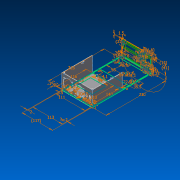
# Autodesk Inventor part: case
Saved by Autodesk Inventor 2015 (Build 190159000, 159)
## iProperties
Created: 2017-03-22
Part Number: case
Material: Generic
Document SubType Name: Modeling
Designer: ZigZagJoe
Density: 1 g/cm^3
Appearance: Default
Author: ZigZagJoe
Autodesk Inventor part; units mm, degrees
ref_plane "YZ Plane" through (0, 0, 0) normal (1, 0, 0) x (0, 1, 0)
ref_plane "XZ Plane" through (0, 0, 0) normal (0, 1, 0) x (-1, 0, 0)
ref_plane "XY Plane" through (0, 0, 0) normal (0, 0, 1) x (1, 0, 0)
sketch "Case Bottom" plane through (0, 0, 0) normal (0, 1, 0) x (-1, 0, 0)
  line L0 (18.5751, 111.0627) -> (-98.4249, 111.0627)
  line L1 (-98.4249, 111.0627) -> (-98.4249, -118.9373)
  line L2 (-98.4249, -118.9373) -> (18.5751, -118.9373)
  line L3 (18.5751, -118.9373) -> (18.5751, 111.0627)
  line L4 (16.5751, 109.0627) -> (-96.4249, 109.0627)
  line L5 (-96.4249, 109.0627) -> (-96.4249, -116.9373)
  line L6 (-96.4249, -116.9373) -> (16.5751, -116.9373)
  line L7 (16.5751, -116.9373) -> (16.5751, 109.0627)
  line L8 (-95.9249, 108.0627) -> (15.0751, 108.0627)
  line L9 (15.0751, 108.0627) -> (15.0751, -106.9373)
  line L10 (15.0751, -106.9373) -> (-95.9249, -106.9373)
  line L11 (-95.9249, -106.9373) -> (-95.9249, 108.0627)
  line L12 (-25.9249, 68.0627) -> (-84.9249, 68.0627)
  line L13 (-84.9249, 68.0627) -> (-84.9249, 15.0627)
  line L14 (-84.9249, 15.0627) -> (-25.9249, 15.0627)
  line L15 (-25.9249, 15.0627) -> (-25.9249, 68.0627)
  line L16 (18.5751, -4.9373) -> (-98.4249, -4.9373)
  line L17 (15.0751, -31.9373) -> (-95.9249, -31.9373)
  circle A0 centre (8.0751, -54.4373) radius 3
  circle A1 centre (8.0751, -54.4373) radius 2.05
  circle A2 centre (-31.4249, -67.4373) radius 3
  circle A3 centre (-31.4249, -67.4373) radius 2.05
  circle A4 centre (-78.3249, -89.9373) radius 3
  circle A5 centre (-78.3249, -89.9373) radius 2.05
  circle A6 centre (-77.9249, -1.9373) radius 3
  circle A7 centre (-77.9249, -1.9373) radius 2.05
  circle A8 centre (8.0751, -4.9373) radius 3
  circle A9 centre (8.5751, 99.0627) radius 3
  circle A10 centre (8.5751, 99.0627) radius 2.05
  circle A11 centre (-33.4249, 100.0627) radius 3
  circle A12 centre (-33.4249, 100.0627) radius 2.05
  circle A13 centre (-88.9249, 82.0627) radius 3
  point P0 (0, 0)
  dimension "d1" = 230
  dimension "d2" = 113
  dimension "d3" = 2
  dimension "d4" = 2
  dimension "d5" = 2
  dimension "d6" = 2
  dimension "d77" = 0.5
  dimension "d78" = 111
  dimension "d79" = 1
  dimension "d129" = 59
  dimension "d130" = 53
  dimension "d131" = 11
  dimension "d132" = 40
  dimension "d181" = 116
  dimension "d200" = 215
  dimension "d201" = 140
  dimension "d202" = 6
  dimension "d203" = 4.1
  dimension "d204" = 22.5
  dimension "d205" = 7
  dimension "d206" = 6
  dimension "d207" = 4.1
  dimension "d208" = 64.5
  dimension "d210" = 35.5
  dimension "d211" = 6
  dimension "d212" = 4.1
  dimension "d213" = 17.6
  dimension "d214" = 58
  dimension "d215" = 6
  dimension "d216" = 4.1
  dimension "d218" = 18
  dimension "d219" = 110
  dimension "d220" = 6
  dimension "d272" = 117
  dimension "d317" = 6
  dimension "d318" = 4.1
  dimension "d319" = 6
  dimension "d320" = 4.1
  dimension "d321" = 6
  dimension "d322" = 26
  dimension "d323" = 7
  dimension "d324" = 62.5
  dimension "d325" = 8
  dimension "d326" = 104.5
  dimension "d327" = 9
  constraints: 36 end point, 14 centre point, 8 parallel, 6 coincident, 6 perpendicular, 5 point on line, 4 horizontal
  measures "d1" distance of L2.end L0.start
  measures "d2" distance of L4.start L4.end
  measures "d3" distance between parallel lines of L3 L7
  measures "d4" distance between parallel lines of L5 L1
  measures "d5" distance between parallel lines of L4 L0
  measures "d6" distance between parallel lines of L2 L6
  measures "d77" distance between parallel lines of L5 L11
  measures "d78" distance of L8.start L8.end
  measures "d79" distance between parallel lines of L8 L4
  measures "d129" distance of L14.end L13.end
  measures "d130" distance of L13.end L12.end
  measures "d131" distance between parallel lines of L11 L13
  measures "d132" distance between parallel lines of L8 L12
  measures "d181" distance between parallel lines of L0 L16
  measures "d200" distance between parallel lines of L10 L8
  measures "d201" distance between parallel lines of L17 L8
  measures "d202" diameter of A0
  measures "d203" diameter of A1
  measures "d204" distance from line of A0.centre L17
  measures "d205" distance from line of L9 A0.centre
  measures "d206" diameter of A2
  measures "d207" diameter of A3
  measures "d208" distance from line of A2.centre L11
  measures "d210" distance from line of A2.centre L17
  measures "d211" diameter of A4
  measures "d212" diameter of A5
  measures "d213" distance from line of L11 A4.centre
  measures "d214" distance from line of L17 A4.centre
  measures "d215" diameter of A6
  measures "d216" diameter of A7
  measures "d218" distance from line of L11 A6.centre
  measures "d219" distance from line of L8 A6.centre
  measures "d220" diameter of A8
  measures "d272" distance between parallel lines of L1 L3
  measures "d317" diameter of A9
  measures "d318" diameter of A10
  measures "d319" diameter of A11
  measures "d320" diameter of A12
  measures "d321" diameter of A13
  measures "d322" distance from line of L8 A13.centre
  measures "d323" distance from line of L11 A13.centre
  measures "d324" distance from line of L11 A11.centre
  measures "d325" distance from line of L8 A11.centre
  measures "d326" distance from line of L11 A9.centre
  measures "d327" distance from line of L8 A9.centre
extrude "Base" add sketch "Case Bottom" along normal blind 3 contours L3 L16 L7 L4 L5 L1 L0 | L3 L2 L1 L16 L5 L6 L7 | L16 L9 L8 L11 L5 L4 L7 | L7 L6 L5 L16 L11 L10 L9 | A6 | L16 A8 L11 L8 L9 | L9 L17 L11 L16 A8 | L9 L10 L11 L17 | A8 L16 | L16 A8 | L15 L14 L13 L12 | A0 | A1 | A2 | A3 | A4 | A5 | A7 | A9 | A10 | A11 | A12 | A13
extrude "Walls" add sketch "Case Bottom" against normal blind 58 contours L3 L16 L7 L4 L5 L1 L0 | L3 L2 L1 L16 L5 L6 L7
sketch "Front Panel" plane through (-18.5751, 3, 111.0627) normal (0, 0, 1) x (1, 0, 0)
  line L0 (113, -51.5) -> (73, -51.5)
  line L1 (73, -51.5) -> (73, -11.5)
  line L2 (73, -11.5) -> (113, -11.5)
  line L3 (113, -11.5) -> (113, -51.5)
  circle A0 centre (109, -47.5) radius 2
  circle A1 centre (77, -47.5) radius 2
  circle A2 centre (77, -15.5) radius 2
  circle A3 centre (109, -15.5) radius 2
  circle A4 centre (93, -31.5) radius 20
  circle A5 centre (109, -47.5) radius 4
  circle A6 centre (109, -15.5) radius 4
  circle A7 centre (77, -15.5) radius 4
  circle A8 centre (77, -47.5) radius 4
  line L4 (115, -3) -> (2, -3) projected
  line L5 (28, -46.875) -> (16, -46.875)
  line L6 (16, -46.875) -> (16, -15.875)
  line L7 (16, -15.875) -> (28, -15.875)
  line L8 (28, -15.875) -> (28, -46.875)
  line L9 (69, -51.5) -> (29, -51.5)
  line L10 (29, -51.5) -> (29, -11.5)
  line L11 (29, -11.5) -> (69, -11.5)
  line L12 (69, -11.5) -> (69, -51.5)
  circle A9 centre (22, -30.5) radius 3.625
  circle A10 centre (22, -39.125) radius 1.5
  circle A11 centre (22, -21.875) radius 1.5
  circle A12 centre (22, -45.375) radius 1.5
  line L13 (2.5, -6.5) -> (114.5, -6.5)
  line L14 (114.5, -6.5) -> (114.5, -7.5)
  line L15 (114.5, -7.5) -> (2.5, -7.5)
  line L16 (2.5, -7.5) -> (2.5, -6.5)
  line L17 (91.5, -9.3) -> (78.5, -9.3)
  line L18 (78.5, -9.3) -> (78.5, -3.3)
  line L19 (78.5, -3.3) -> (91.5, -3.3)
  line L20 (91.5, -3.3) -> (91.5, -9.3)
  line L21 (68.5, -8.7) -> (63.5, -8.7)
  line L22 (62.5, -7.7) -> (62.5, -4.7)
  line L23 (62.5, -4.7) -> (69.5, -4.7)
  line L24 (69.5, -4.7) -> (69.5, -7.7)
  arc A13 (68.5, -8.7) -> (69.5, -7.7) centre (68.5, -7.7) ccw
  arc A14 (62.5, -7.7) -> (63.5, -8.7) centre (63.5, -7.7) ccw
  circle A15 centre (12, -6.75) radius 0.6
  line L25 (115, -3) -> (115, -61) projected
  line L26 (2, -3) -> (2, -61) projected
  line L27 (15, -11.5) -> (2.5, -11.5)
  line L28 (2.5, -11.5) -> (2.5, -49.5)
  line L29 (2.5, -49.5) -> (15, -49.5)
  line L30 (15, -49.5) -> (15, -11.5)
  line L31 (117, -61) -> (0, -61) projected
  line L32 (0, 0) -> (117, 0) projected
  line L33 (12.25, -37.5) -> (5.25, -37.5)
  line L34 (5.25, -37.5) -> (5.25, -23.5)
  line L35 (5.25, -23.5) -> (12.25, -23.5)
  line L36 (12.25, -23.5) -> (12.25, -37.5)
  circle A16 centre (8.75, -45) radius 1.6
  circle A17 centre (8.75, -16) radius 1.6
  point P0 (18.5751, -3)
  point P1 (62.5, -8.7)
  dimension "d11" = 40
  dimension "d12" = 40
  dimension "d13" = 4
  dimension "d14" = 4
  dimension "d15" = 4
  dimension "d16" = 4
  dimension "d17" = 32
  dimension "d18" = 32
  dimension "d19" = 32
  dimension "d20" = 32
  dimension "d21" = 4
  dimension "d22" = 4
  dimension "d23" = 40
  dimension "d31" = 2
  dimension "d32" = 8.5
  dimension "d33" = 4
  dimension "d34" = 8
  dimension "d35" = 20
  dimension "d36" = 20
  dimension "d37" = 12
  dimension "d38" = 31
  dimension "d39" = 40
  dimension "d40" = 4
  dimension "d41" = 7.25
  dimension "d42" = 3
  dimension "d43" = 3
  dimension "d44" = 8.625
  dimension "d45" = 8.625
  dimension "d46" = 6
  dimension "d47" = 6
  dimension "d48" = 0
  dimension "d49" = 0
  dimension "d50" = 6
  dimension "d51" = 3
  dimension "d52" = 6.25
  dimension "d53" = 0
  dimension "d59" = 112
  dimension "d60" = 1
  dimension "d61" = 3.5
  dimension "d62" = 13
  dimension "d63" = 6
  dimension "d64" = 7
  dimension "d65" = 4
  dimension "d66" = 1.8
  dimension "d67" = 3.2
  dimension "d68" = 23
  dimension "d69" = 45
  dimension "d70" = 1
  dimension "d71" = 1.2
  dimension "d72" = 102.5
  dimension "d73" = 0.75
  dimension "d74" = 0.5
  dimension "d275" = 12.5
  dimension "d276" = 38
  dimension "d277" = 30.5
  dimension "d278" = 61
  dimension "d279" = 3.2
  dimension "d280" = 3.2
  dimension "d281" = 3.5
  dimension "d282" = 7
  dimension "d283" = 14
  dimension "d285" = 7.5
  dimension "d286" = 3.5
  dimension "d287" = 29
  constraints: 64 end point, 18 centre point, 16 parallel, 8 horizontal, 8 perpendicular, 8 tangent, 4 coincident, 4 point on circle, 2 point on line, 1 equal radius
  measures "d11" distance of L1.end L2.end
  measures "d12" distance of L0.end L1.end
  measures "d13" diameter of A0
  measures "d14" diameter of A1
  measures "d15" diameter of A2
  measures "d16" diameter of A3
  measures "d17" distance of A0.centre A3.centre
  measures "d18" distance of A1.centre A0.centre
  measures "d19" distance of A1.centre A2.centre
  measures "d20" distance of A3.centre A2.centre
  measures "d21" distance from line of L0 A0.centre
  measures "d22" distance from line of L3 A0.centre
  measures "d23" diameter of A4
  measures "d31" horizontal distance of L0.start L4.start
  measures "d32" distance between parallel lines of L4 L2
  measures "d33" distance from line of L1 A2.centre
  measures "d34" diameter of A7
  measures "d35" distance from line of L3 A4.centre
  measures "d36" distance from line of A4.centre L2
  measures "d37" distance of L6.end L7.end
  measures "d38" distance of L5.end L6.end
  measures "d39" distance of L10.end L11.end
  measures "d40" distance between parallel lines of L12 L1
  measures "d41" diameter of A9
  measures "d42" diameter of A10
  measures "d43" diameter of A11
  measures "d44" distance of A9.centre A11.centre
  measures "d45" distance of A9.centre A10.centre
  measures "d46" distance from line of L8 A9.centre
  measures "d47" distance from line of L6 A9.centre
  measures "d48" horizontal distance of A9.centre A10.centre
  measures "d49" horizontal distance of A9.centre A11.centre
  measures "d50" distance from line of L7 A11.centre
  measures "d51" diameter of A12
  measures "d52" distance of A12.centre A10.centre
  measures "d53" horizontal distance of A12.centre A10.centre
  measures "d59" distance of L14.end L15.end
  measures "d60" distance of L13.end L14.end
  measures "d61" distance between parallel lines of L4 L13
  measures "d62" distance of L18.end L19.end
  measures "d63" distance of L17.end L18.end
  measures "d64" distance of L22.end L23.end
  measures "d65" distance of point (62.5, -8.7) L22.end
  measures "d66" distance between parallel lines of L13 L23
  measures "d67" distance between parallel lines of L13 L19
  measures "d68" distance between parallel lines of L20 L14
  measures "d69" distance between parallel lines of L24 L14
  measures "d70" radius of A13
  measures "d71" diameter of A15
  measures "d72" distance from line of L14 A15.centre
  measures "d73" distance from line of L15 A15.centre
  measures "d74" distance between parallel lines of L25 L14
  measures "d275" distance of L27.start L27.end
  measures "d276" distance between parallel lines of L29 L27
  measures "d277" distance from line of L31 A9.centre
  measures "d278" distance between parallel lines of L31 L32
  measures "d279" diameter of A16
  measures "d280" diameter of A17
  measures "d281" distance from line of L34 A17.centre
  measures "d282" distance between parallel lines of L34 L36
  measures "d283" distance of L35.end L33.start
  measures "d285" distance from line of L35 A17.centre
  measures "d286" distance from line of A16.centre L34
  measures "d287" distance of A17.centre A16.centre
sketch "Rear Panel" plane through (98.4249, 3, -118.9373) normal (0, 0, -1) x (-1, 0, 0)
  line L0 (68.5, -51) -> (14.5, -51)
  line L1 (14.5, -51) -> (14.5, -39)
  line L2 (14.5, -39) -> (68.5, -39)
  line L3 (68.5, -39) -> (68.5, -51)
  circle A0 centre (75, -45) radius 1.5
  circle A1 centre (8, -45) radius 1.5
  line L4 (78.5, -56) -> (4.5, -56)
  line L5 (4.5, -56) -> (4.5, -34)
  line L6 (4.5, -34) -> (78.5, -34)
  line L7 (78.5, -34) -> (78.5, -56)
  line L8 (91.5, -33) -> (3.5, -33)
  line L9 (3.5, -33) -> (3.5, -58)
  line L10 (3.5, -58) -> (91.5, -58)
  line L11 (91.5, -58) -> (91.5, -33)
  line L12 (0, -61) -> (0, 0) projected
  line L13 (115, -16) -> (79.4, -16)
  line L14 (79.4, -16) -> (79.4, -53)
  line L15 (79.4, -53) -> (115, -53)
  line L16 (115, -53) -> (115, -16)
  circle A2 centre (83.4, -20) radius 1.75
  circle A3 centre (83.4, -49) radius 1.75
  line L17 (115, -53) -> (87, -53)
  line L18 (87, -53) -> (87, -16)
  line L19 (87, -16) -> (115, -16)
  line L20 (115, -16) -> (115, -53)
  line L21 (110, -46) -> (94, -46)
  line L22 (94, -46) -> (94, -25)
  line L23 (94, -25) -> (110, -25)
  line L24 (110, -25) -> (110, -46)
  line L25 (2.5, -6.5) -> (114.5, -6.5)
  line L26 (114.5, -6.5) -> (114.5, -7.5)
  line L27 (114.5, -7.5) -> (2.5, -7.5)
  line L28 (2.5, -7.5) -> (2.5, -6.5)
  line L29 (2, -3) -> (2, -61) projected
  line L30 (115, -3) -> (2, -3) projected
  line L31 (114.5, -7.5) -> (94.5, -7.5)
  line L32 (94.5, -7.5) -> (94.5, -14)
  line L33 (94.5, -14) -> (114.5, -14)
  line L34 (114.5, -14) -> (114.5, -7.5)
  line L35 (72.8, -28.695) -> (74.8, -27.5403)
  line L36 (74.8, -27.5403) -> (76.8, -28.695)
  line L37 (76.8, -28.695) -> (76.8, -31.0044)
  line L38 (76.8, -31.0044) -> (74.8, -32.1591)
  line L39 (74.8, -32.1591) -> (72.8, -31.0044)
  line L40 (72.8, -31.0044) -> (72.8, -28.695)
  line L41 (70, -23.8453) -> (72, -22.6906)
  line L42 (72, -22.6906) -> (74, -23.8453)
  line L43 (74, -23.8453) -> (74, -26.1547)
  line L44 (74, -26.1547) -> (72, -27.3094)
  line L45 (72, -27.3094) -> (70, -26.1547)
  line L46 (70, -26.1547) -> (70, -23.8453)
  line L47 (117, -61) -> (117, 0) projected
  line L48 (103.6, -55.0359) -> (105.6, -53.8812)
  line L49 (105.6, -53.8812) -> (107.6, -55.0359)
  line L50 (107.6, -55.0359) -> (107.6, -57.3453)
  line L51 (107.6, -57.3453) -> (105.6, -58.5)
  line L52 (105.6, -58.5) -> (103.6, -57.3453)
  line L53 (103.6, -57.3453) -> (103.6, -55.0359)
  line L54 (103.6, -14.3448) -> (105.6, -13.1901)
  line L55 (105.6, -13.1901) -> (107.6, -14.3448)
  line L56 (107.6, -14.3448) -> (107.6, -16.6542)
  line L57 (107.6, -16.6542) -> (105.6, -17.8089)
  line L58 (105.6, -17.8089) -> (103.6, -16.6542)
  line L59 (103.6, -16.6542) -> (103.6, -14.3448)
  line L60 (100.8, -9.495) -> (102.8, -8.3403)
  line L61 (102.8, -8.3403) -> (104.8, -9.495)
  line L62 (104.8, -9.495) -> (104.8, -11.8044)
  line L63 (104.8, -11.8044) -> (102.8, -12.9591)
  line L64 (102.8, -12.9591) -> (100.8, -11.8044)
  line L65 (100.8, -11.8044) -> (100.8, -9.495)
  line L66 (103.6, -4.6453) -> (105.6, -3.4906)
  line L67 (105.6, -3.4906) -> (107.6, -4.6453)
  line L68 (107.6, -4.6453) -> (107.6, -6.9547)
  line L69 (107.6, -6.9547) -> (105.6, -8.1094)
  line L70 (105.6, -8.1094) -> (103.6, -6.9547)
  line L71 (103.6, -6.9547) -> (103.6, -4.6453)
  line L72 (115, -3) -> (115, -61) projected
  line L73 (117, -61) -> (0, -61) projected
  line L74 (84.1, -49) -> (82.7, -49) construction
  line L75 (84.1, -47.25) -> (82.7, -47.25)
  line L76 (82.7, -50.75) -> (84.1, -50.75)
  arc A4 (84.1, -50.75) -> (84.1, -47.25) centre (84.1, -49) ccw
  arc A5 (82.7, -47.25) -> (82.7, -50.75) centre (82.7, -49) ccw
  line L77 (84.1, -20) -> (82.7, -20) construction
  line L78 (84.1, -18.25) -> (82.7, -18.25)
  line L79 (82.7, -21.75) -> (84.1, -21.75)
  arc A6 (84.1, -21.75) -> (84.1, -18.25) centre (84.1, -20) ccw
  arc A7 (82.7, -18.25) -> (82.7, -21.75) centre (82.7, -20) ccw
  line L80 (83.4, -20) -> (84.8, -20) construction
  line L81 (0, 0) -> (117, 0) projected
  line L82 (117, 0) -> (117, -61) projected
  line L83 (117, -1) -> (0, -1)
  circle A8 centre (83.4, -20) radius 3.1976
  point P0 (98.4249, -3)
  point P1 (74.8, -29.8497)
  point P2 (72, -25)
  point P3 (105.6, -56.1906)
  point P4 (105.6, -15.4995)
  point P5 (102.8, -10.6497)
  point P6 (105.6, -5.8)
  dimension "d80" = 3
  dimension "d81" = 3
  dimension "d83" = 54
  dimension "d84" = 6.5
  dimension "d85" = 6.5
  dimension "d86" = 10
  dimension "d87" = 10
  dimension "d88" = 11
  dimension "d89" = 5
  dimension "d90" = 5
  dimension "d91" = 2
  dimension "d92" = 1
  dimension "d93" = 13
  dimension "d94" = 1
  dimension "d96" = 12
  dimension "d97" = 22
  dimension "d100" = 3
  dimension "d105" = 35.6
  dimension "d106" = 37
  dimension "d107" = 3.5
  dimension "d108" = 3.5
  dimension "d109" = 4
  dimension "d110" = 4
  dimension "d111" = 4
  dimension "d112" = 4
  dimension "d113" = 28
  dimension "d115" = 21
  dimension "d116" = 7
  dimension "d117" = 9
  dimension "d118" = 0
  dimension "d119" = 8
  dimension "d120" = 112
  dimension "d121" = 1
  dimension "d122" = 0.5
  dimension "d123" = 3.5
  dimension "d124" = 6.5
  dimension "d139" = 4
  dimension "d140" = 4
  dimension "d150" = 1.6
  dimension "d151" = 0.8
  dimension "d152" = 6.8
  dimension "d153" = 9.4685
  dimension "d154" = 4
  dimension "d165" = 4
  dimension "d166" = 4
  dimension "d167" = 1.6
  dimension "d168" = 0.8
  dimension "d169" = 6.8
  dimension "d170" = 9.4685
  dimension "d171" = 1.6
  dimension "d172" = 4
  dimension "d178" = 2.8
  dimension "d179" = 9.4
  dimension "d187" = 29
  dimension "d188" = 12
  dimension "d194" = 31.6
  dimension "d195" = 0.7
  dimension "d196" = 0.7
  dimension "d197" = 180
  dimension "d299" = 2.5
  dimension "d300" = 0.8
  dimension "d301" = 25
  dimension "d302" = 45
  dimension "d303" = 41
  constraints: 156 end point, 25 parallel, 11 horizontal, 9 centre point, 9 perpendicular, 8 point on circle, 8 tangent, 3 point on line, 2 midpoint, 1 coincident, 1 collinear, 78 other
  measures "d80" diameter of A0
  measures "d81" diameter of A1
  measures "d83" distance of L1.end L2.end
  measures "d84" distance from line of L3 A0.centre
  measures "d85" distance from line of A1.centre L1
  measures "d86" distance between parallel lines of L3 L7
  measures "d87" distance between parallel lines of L5 L1
  measures "d88" distance from line of L4 A0.centre
  measures "d89" distance between parallel lines of L4 L0
  measures "d90" distance between parallel lines of L6 L2
  measures "d91" distance between parallel lines of L10 L4
  measures "d92" distance between parallel lines of L6 L8
  measures "d93" distance between parallel lines of L11 L7
  measures "d94" distance between parallel lines of L9 L5
  measures "d96" distance of L2.end L0.start
  measures "d97" distance between parallel lines of L4 L6
  measures "d100" vertical distance of L12.start L9.end
  measures "d105" distance of L15.end L14.end
  measures "d106" distance of L14.end L13.end
  measures "d107" diameter of A2
  measures "d108" diameter of A3
  measures "d109" distance from line of L14 L80.start
  measures "d110" distance from line of L13 L80.start
  measures "d111" distance from line of L15 A3.centre
  measures "d112" distance from line of L14 A3.centre
  measures "d113" distance of L18.end L19.end
  measures "d115" distance between parallel lines of L22 L16
  measures "d116" distance between parallel lines of L15 L21
  measures "d117" distance between parallel lines of L13 L23
  measures "d118" distance from line of L72.end L16
  measures "d119" distance from line of L72.end L17
  measures "d120" distance of L26.end L27.end
  measures "d121" distance of L25.end L26.end
  measures "d122" distance from line of L29 L25.start
  measures "d123" distance between parallel lines of L25 L30
  measures "d124" distance of L32.end L31.end
  measures "d139" distance between parallel lines of L37 L40
  measures "d140" distance between parallel lines of L46 L43
  measures "d150" distance between parallel lines of L44 L35
  measures "d151" horizontal distance of L43.end L35.end
  measures "d152" horizontal distance of L45.end L36.end
  measures "d153" vertical distance of L41.end L38.end
  measures "d154" distance between parallel lines of L50 L53
  measures "d165" distance between parallel lines of L56 L59
  measures "d166" distance between parallel lines of L65 L62
  measures "d167" distance between parallel lines of L63 L54
  measures "d168" horizontal distance of L62.end L54.end
  measures "d169" horizontal distance of L64.end L55.end
  measures "d170" vertical distance of L61.start L57.end
  measures "d171" distance between parallel lines of L61 L70
  measures "d172" distance between parallel lines of L69 L66
  measures "d178" distance from line of L30 point (105.6, -5.8)
  measures "d179" distance from line of L72 point (105.6, -5.8)
  measures "d187" distance of L80.start A3.centre
  measures "d188" distance from line of L73 A3.centre
  measures "d194" distance from line of A3.centre L72
  measures "d195" distance of A3.centre L74.end
  measures "d196" distance of L80.start L77.end
  measures "d197" angle of L77 L80
  measures "d299" distance from line of L73 L51.end
  measures "d300" distance from line of L62 L69.end
  measures "d301" distance from line of L81 point (72, -25)
  measures "d302" distance from line of point (72, -25) L47
  measures "d303" distance from line of L73 L80.start
extrude "Fan Cutout" cut sketch "Front Panel" against normal blind 2 contours A4 A8 A7 A6 A5 | A5 A4 | A4 A8 | A6 A4 | A4 A7 | A0 | A1 | A2 | A3 picked at (106.7084, -45.4196) picked at (79.0804, -45.2084) picked at (106.7084, -17.5804) picked at (79.0804, -17.7916)
extrude "Fan Hole Supports" add sketch "Front Panel" against normal blind 2 contours A5 A4 | A5 A4 | A8 A4 | A4 A8 | A6 A4 | A6 A4 | A7 A4 | A4 A7
pattern_linear "Fan Two" count 2 spacing 44 along (-1, 0, 0) of "Fan Hole Supports", "Fan Cutout"
extrude "Power Button Cutout" cut sketch "Front Panel" against normal blind 2 contours A12 | A9 | A10 | A11
extrude "Power LED Cover" add sketch "Front Panel" against normal blind 1 contours A12
extrude "Mobo Ports Cutout" cut sketch "Front Panel" against normal blind 2 contours A15 L13 | L13 A15 | L22 L13 L24 L15 | L15 L24 A13 L21 A14 L22 | L22 L23 L24 L13 | L18 L13 L20 L15 | L15 L20 L17 L18 | L18 L19 L20 L13
extrude "USB Panel mount cutout" cut sketch "Front Panel" against normal blind 2 contours L33 L34 L35 L36 | A16 | A17
sketch "Cover screw mounts" plane through (0, -58, 0) normal (0, -1, 0) x (1, 0, 0)
  line L0 (-16.5751, -116.9373) -> (-16.5751, 109.0627) projected
  line L1 (-18.5751, 111.0627) -> (-18.5751, -118.9373) projected
  line L2 (98.4249, -118.9373) -> (98.4249, 111.0627) projected
  circle A0 centre (95.4249, -115.9373) radius 2.05
  circle A1 centre (95.4249, -115.9373) radius 3
  line L3 (-18.5751, -118.9373) -> (98.4249, -118.9373) projected
  point P0 (-16.5751, 108.0627)
  dimension "d248" = 4.1
  dimension "d249" = 6
  dimension "d267" = 3
  dimension "d268" = 3
  constraints: 2 centre point, 2 coincident
  measures "d248" diameter of A0
  measures "d249" diameter of A1
  measures "d267" distance from line of L3 A0.centre
  measures "d268" distance from line of L2 A0.centre
extrude "NIC Mount" cut sketch "Rear Panel" against normal blind 2 contours L0 L1 L2 L3 | A0 | A1
extrude "PSU Mount (Rear)" cut sketch "Rear Panel" against normal blind 2 contours A2 | A3 | L21 L22 L23 L24
sketch "Sketch5" plane through (-18.5751, 3, -118.9373) normal (-1, 0, 0) x (0, 0, 1)
  circle A0 centre (99, -49) radius 1.5
  circle A1 centre (99, -20) radius 1.5
  line L0 (2, -61) -> (228, -61) projected
  line L1 (2, -3) -> (2, -61) projected
  line L2 (99.7, -49) -> (98.3, -49) construction
  line L3 (99.7, -47.5) -> (98.3, -47.5)
  line L4 (98.3, -50.5) -> (99.7, -50.5)
  arc A2 (99.7, -50.5) -> (99.7, -47.5) centre (99.7, -49) ccw
  arc A3 (98.3, -47.5) -> (98.3, -50.5) centre (98.3, -49) ccw
  line L5 (99.7, -20) -> (98.3, -20) construction
  line L6 (99.7, -18.5858) -> (98.3, -18.5858)
  line L7 (98.3, -21.4142) -> (99.7, -21.4142)
  arc A4 (99.7, -21.4142) -> (99.7, -18.5858) centre (99.7, -20) ccw
  arc A5 (98.3, -18.5858) -> (98.3, -21.4142) centre (98.3, -20) ccw
  point P0 (118.9373, -3)
  dimension "d184" = 3
  dimension "d185" = 3
  dimension "d186" = 29
  dimension "d189" = 12
  dimension "d190" = 0
  dimension "d191" = 97
  dimension "d198" = 0.7
  dimension "d199" = 0.7
  dimension "d304" = 41
  constraints: 16 end point, 8 point on circle, 8 tangent, 6 centre point, 2 horizontal, 2 midpoint, 2 parallel
  measures "d184" diameter of A0
  measures "d185" diameter of A1
  measures "d186" distance of A0.centre A1.centre
  measures "d189" distance from line of L0 A0.centre
  measures "d190" horizontal distance of A1.centre A0.centre
  measures "d191" distance from line of L1 A0.centre
  measures "d198" distance of A0.centre L2.end
  measures "d199" distance of A1.centre L5.end
  measures "d304" distance from line of L0 A1.centre
extrude "PSU Mount (Side)" cut sketch "Sketch5" against normal blind 3 contours A0 | A1 L7 L6 | L6 A1 | A1 L7
extrude "Hex Vent Main" cut sketch "Rear Panel" against normal blind 2 contours L35 L36 L37 L38 L39 L40 | L41 L42 L43 L44 L45 L46
pattern_linear "Hex Vent Main Pattern" count 13 spacing 5.6 along (1, 0, 0) count 3 spacing 9.6 along (0, 1, 0) of "Hex Vent Main"
extrude "Hex Vent PSU Upper" cut sketch "Rear Panel" against normal blind 2 contours L48 L49 L50 L51 L52 L53
pattern_linear "Hex Vent PSU Upper Pattern" count 7 spacing 5.6 along (1, 0, 0) of "Hex Vent PSU Upper"
extrude "Hex Vent PSU Lower" cut sketch "Rear Panel" against normal blind 2 contours L59 L54 L33 L55 L56 L13 | L13 L56 L57 L58 L59 | L54 L55 L33 | L70 L71 L25 L68 L69 L27 | L27 L69 L70 | L25 L71 L66 L67 L68 | L60 L61 L62 L63 L64 L65
pattern_linear "Hex Vent PSU Lower Pattern" count 7 spacing 5.6 along (1, 0, 0) of "Hex Vent PSU Lower"
extrude "Top Screw Mounts" add sketch "Cover screw mounts" against normal blind 4.5 contours A1
sketch "Reolve Sketch" plane through (96.4249, -58, 109.0627) normal (-1, 0, 0) x (0, 0, 1)
  line L0 (-225, 12.7424) -> (-225, 0)
  line L1 (-225, 0) -> (-222.1716, 0)
  line L2 (-222.1716, 0) -> (-222.1716, 4.9714)
  line L3 (-222.1716, 4.9714) -> (-225, 12.7424)
  line L4 (-228, 0) -> (-228, 61) projected
  point P0 (-109.0627, 58)
  dimension "d269" = 20
  dimension "d270" = 3
  constraints: 8 end point, 2 perpendicular
  measures "d269" angle of L0 L3
  measures "d270" distance between parallel lines of L4 L0
revolve "Screw Mount Support" [suppressed]
extrude "Screw mount cutout" cut sketch "Cover screw mounts" against normal blind 3.5 contours A0
pattern_linear "Screw Mount Pattern" count 4 spacing 74.66 along (0, 0, 1) count 2 spacing 111 along (-1, 0, 0) of "Screw mount cutout", "Top Screw Mounts"
fillet "Screw Mount Fillet" radius 3 16 edges at (96.4249, -55.75, -38.4488) (96.4249, -55.75, 36.2112) (96.4249, -55.75, -113.1088) (96.4249, -55.75, -44.1057) (96.4249, -55.75, 30.5543) (96.4249, -55.75, 105.2143) (92.6037, -55.75, 109.0627) (-16.5751, -55.75, 30.5543) (-16.5751, -55.75, 36.2112) (-12.7538, -55.75, 109.0627) (-16.5751, -55.75, 105.2143) (-16.5751, -55.75, -38.4488) (-16.5751, -55.75, -44.1057) (-16.5751, -55.75, -113.1088) (-12.7466, -55.75, -116.9373) (92.5965, -55.75, -116.9373)
fillet "Exterior Fillet" [suppressed]
fillet "Interior Fillet" radius 1 8 edges at (96.4249, -27.25, -116.9373) (96.4249, -27.25, 109.0627) (96.4249, 0, -3.9373) (39.9249, 0, 109.0627) (-16.5751, 0, -3.9373) (39.9249, 0, -116.9373) (-16.5751, -27.25, -116.9373) (-16.5751, -27.25, 109.0627)
extrude "2mm bottom HACK" cut sketch "Rear Panel" against normal blind 240 contours L83 L12 L81 L47
fillet "Bottom fillet" radius 1 2 edges at (-18.5751, 2, -3.9373) (98.4249, 2, -3.9373)
fillet "Top fillet (for print quality)" radius 0.2 29 edges at (-18.5751, -58, 109.5527) (-18.5751, -58, 70.7127) (-18.5751, -58, -3.9473) (-18.5751, -58, -78.6073) (-18.5751, -58, -117.4373) (-12.5751, -58, -41.2773) (-16.0246, -58, -45.2021) (-16.5751, -58, -78.6073) (-16.0246, -58, -112.0125) (-13.4537, -58, -113.8159) (-11.6503, -58, -116.3868) (39.9249, -58, -116.9373) (91.5001, -58, -116.3868) (93.3036, -58, -113.8159) (95.8744, -58, -112.0125) (96.4249, -58, -78.6073) (95.8744, -58, -45.2021) (92.4249, -58, -41.2773) (95.8744, -58, -37.3525) (96.4249, -58, 70.7127) (96.4249, -58, -3.9473) (-16.5751, -58, -3.9473) (-16.5751, -58, 70.7127) (-16.0246, -58, -37.3525) (98.4249, -58, 109.5527) (98.4249, -58, 70.7127) (98.4249, -58, -117.4373) (98.4249, -58, -3.9473) (98.4249, -58, -78.6073)
extrude "PSU Mounting hole protection" add sketch "Rear Panel" against normal blind 2 contours A8
extrude "Standoffs" add sketch "Case Bottom" against normal blind 3.5 contours A6 | A8 L16 | L16 A8 | A0 | A2 | A4 | A9 | A11 | A13
fillet "Standoffs Fillet" radius 2 8 edges at (81.3249, 0, -89.9373) (34.4249, 0, -67.4373) (80.9249, 0, -1.9373) (91.9249, 0, 82.0627) (36.4249, 0, 100.0627) (-5.5751, 0, 99.0627) (-5.0751, 0, -4.9373) (-5.0751, 0, -54.4373)
extrude "Sectioning Cut (front only)" cut sketch "Case Bottom" along normal mid plane 200 contours L3 L2 L1 L16 L5 L6 L7 | L7 L6 L5 L16 L11 L10 L9 | L9 L17 L11 L16 A8 | L9 L10 L11 L17 | A8 L16 | A0 | A1 | A2 | A3 | A4 | A5 picked at (8.9896, -5.6413)
extrude "Sectioning Cut (rear only)" [suppressed]
equation "\"d13\" = d16"
equation "\"d14\" = d16"
equation "\"d15\" = d16"
equation "\"d45\" = d44"
equation "\"d46\" = d47"
equation "\"d88\" = 0.5 * d97"
equation "\"d140\" = d139"
body "Solid1"
body "Solid2"
body "Solid3"
body "Solid4"
body "Solid5"
body "Solid6"
